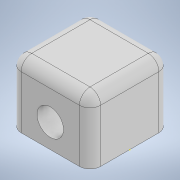
# Autodesk Inventor part: Connector
Saved by Autodesk Inventor 2021 (Build 250183000, 183)
## iProperties
Created: 2021-02-05
Part Number: Connector
Material: Generic
Document SubType Name: Modeling
Designer: nevkd
Density: 1 g/cm^3
Appearance: Default
Mass: 2.31812 g
Surface Area: 12.6794 cm^2
Volume: 2.31812 cm^3
Author: nevkd
Autodesk Inventor part; units mm, degrees
ref_plane "YZ Plane" through (0, 0, 0) normal (1, 0, 0) x (0, 1, 0)
ref_plane "XZ Plane" through (0, 0, 0) normal (0, 1, 0) x (-1, 0, 0)
ref_plane "XY Plane" through (0, 0, 0) normal (0, 0, 1) x (1, 0, 0)
sketch "Sketch1" plane through (0, 0, 0) normal (0, 1, 0) x (-1, 0, 0)
  point P0 (0, 0)
sketch "Sketch2" plane through (0, 0, 0) normal (0, 1, 0) x (-1, 0, 0)
  line L0 (0, 0) -> (0, -7.5)
  line L1 (0, 0) -> (0, 7.5)
  line L2 (0, 7.5) -> (15, 7.5)
  line L3 (0, -7.5) -> (15, -7.5)
  line L4 (15, -7.5) -> (15, 7.5)
  dimension "d0" = 7.5
  dimension "d1" = 7.5
  dimension "d2" = 15
  constraints: 10 end point, 2 horizontal, 2 vertical, 1 perpendicular
  measures "d0" distance of L0.start L0.end
  measures "d1" distance of L0.start L1.end
  measures "d2" distance of L1.end L2.end
extrude "Extrusion1" add sketch "Sketch2" along normal blind 12
sketch "Sketch3" plane through (-15, 0, 7.5) normal (0, 0, 1) x (1, 0, 0)
  line L0 (0, 0) -> (0, 12) projected
  circle A0 centre (7.5, 4.5) radius 2.5
  line L1 (0, 12) -> (15, 12) projected
  point P0 (15, 0)
  dimension "d6" = 5
  dimension "d12" = 7.5
  constraints: 1 centre point
  measures "d6" diameter of A0
  measures "d12" distance from line of L1 A0.centre
fillet "Fillet1" radius 2 4 edges at (0, 12, -3.75) (-15, 12, 0) (-7.5, 12, 7.5) (-7.5, 12, -7.5)
extrude "Extrusion2" cut sketch "Sketch3" against normal blind 15
fillet "Fillet2" radius 2 6 edges at (-14.4142, 11.4142, 6.9142) (-15, 5, 7.5) (-0.5858, 11.4142, 6.9142) (0, 5, 7.5) (-14.4142, 11.4142, -6.9142) (-15, 5, -7.5)
fillet "Fillet3" radius 2 2 edges at (-0.5858, 11.4142, -6.9142) (0, 5, -7.5)
body "Solid1"
